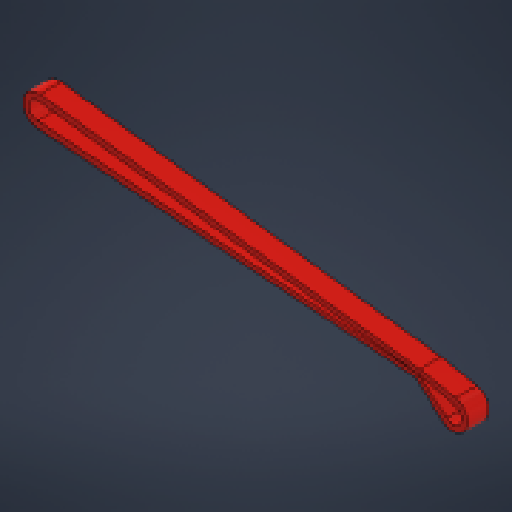
# Autodesk Inventor part: Angel Changer left band up
Saved by Autodesk Inventor 2023.2 (Build 272271030, 271C)
## iProperties
Created: 2023-04-07
Part Number: Angel Changer left band up
Material: Generic
Document SubType Name: Modeling
Designer: Main Account
Density: 1 g/cm^3
Appearance: Default
Author: Main Account
Autodesk Inventor part; units mm, degrees
ref_plane "YZ Plane" through (0, 0, 0) normal (1, 0, 0) x (0, 1, 0)
ref_plane "XZ Plane" through (0, 0, 0) normal (0, 1, 0) x (-1, 0, 0)
ref_plane "XY Plane" through (0, 0, 0) normal (0, 0, 1) x (1, 0, 0)
sketch "Sketch1" plane through (0, 0, 0) normal (0, 0, 1) x (1, 0, 0)
  circle A0 centre (5.9832, 5.1816) radius 4.191 construction
  line L0 (94.1996, -4.6837) -> (92.7687, -5.3712) construction
  circle A1 centre (102.6732, -7.6575) radius 2.1844 construction
  arc A2 (101.3367, -9.255) -> (103.1438, -5.6286) centre (102.6732, -7.6575) ccw
  arc A3 (6.2383, 7.2488) -> (5.8246, 3.1049) centre (5.9832, 5.1816) ccw
  arc A4 (6.4347, 8.7359) -> (5.7291, 1.6079) centre (5.9832, 5.1816) ccw
  arc A5 (100.2365, -10.2841) -> (103.3582, -4.1408) centre (102.6732, -7.6575) ccw
  line L1 (100.2365, -10.2841) -> (94.1996, -4.6837)
  line L2 (101.3367, -9.255) -> (94.6775, -3.6837)
  line L3 (5.8246, 3.1049) -> (94.6775, -3.6837)
  line L4 (94.1996, -4.6837) -> (5.7291, 1.6079)
  line L5 (103.1438, -5.6286) -> (94.6857, -3.6666)
  line L6 (94.6857, -3.6666) -> (6.2383, 7.2488)
  line L7 (6.4347, 8.7359) -> (95.0262, -2.5179)
  line L8 (95.0262, -2.5179) -> (103.3582, -4.1408)
  line L9 (94.1996, -4.6837) -> (94.6775, -3.6837) construction
  point P0 (0, 0)
  dimension "d0" = 4.1656
  dimension "d1" = 4.1656
  dimension "d2" = 1.5
  dimension "d3" = 1.5
  dimension "d4" = 1
  dimension "d5" = 2.666
  constraints: 19 end point, 8 point on circle, 8 tangent, 4 centre point, 2 coincident, 1 other
  measures "d0" diameter of A2
  measures "d1" diameter of A3
  measures "d2" radial gap between concentric circles of A3 A4
  measures "d3" radial gap between concentric circles of A2 A5
  measures "d4" vertical distance of L0.start L2.end
  measures "d5" angle of L6 L3
extrude "Extrusion1" add sketch "Sketch1" along normal blind 5
body "Solid1"
